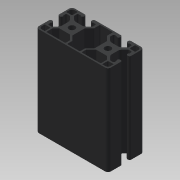
# Autodesk Inventor part: 40-4084-LITE-BLACK-FB
Saved by Autodesk Inventor 2013 (Build 170138000, 138)
## iProperties
Company: 80/20 Inc.
Created: 2014-04-23
Part Number: 40-4084-LITE-BLACK-FB
Material: Generic
Document SubType Name: Modeling
Designer: Ross Bowman
Density: 1 g/cm^3
Engineer: Ross Bowman
Catalog Web Link: 8020.net
Vendor: 80/20 Inc.
Material: 6105-T5 Aluminum
Author: Ross Bowman
Keywords: 80/20 , 8020 , T-Slot , Extrusion
Autodesk Inventor part; units mm, degrees
ref_plane "YZ Plane" through (0, 0, 0) normal (1, 0, 0) x (0, 1, 0)
ref_plane "XZ Plane" through (0, 0, 0) normal (0, 1, 0) x (-1, 0, 0)
ref_plane "XY Plane" through (0, 0, 0) normal (0, 0, 1) x (1, 0, 0)
sketch "Sketch1" plane through (0, 0, 0) normal (0, 0, 1) x (1, 0, 0)
  arc A0 (32.3165, 18.3492) -> (31.9365, 17.9693) centre (32.3165, 17.9693) ccw
  line L0 (35.5555, 18.3492) -> (32.3165, 18.3492)
  arc A1 (38.3495, 15.5552) -> (35.5555, 18.3492) centre (35.5555, 15.5552) ccw
  line L1 (38.3495, 12.3165) -> (38.3495, 15.5552)
  arc A2 (37.9695, 11.9365) -> (38.3495, 12.3165) centre (37.9695, 12.3165) ccw
  line L2 (33.2063, 11.9365) -> (37.9695, 11.9365)
  arc A3 (31.9365, 13.2063) -> (33.2063, 11.9365) centre (33.2063, 13.2063) ccw
  line L3 (31.9365, 17.9693) -> (31.9365, 13.2063)
  arc A4 (35.5555, -18.3492) -> (38.3495, -15.5552) centre (35.5555, -15.5552) ccw
  line L4 (32.3165, -18.3492) -> (35.5555, -18.3492)
  arc A5 (31.9365, -17.9693) -> (32.3165, -18.3492) centre (32.3165, -17.9693) ccw
  line L5 (31.9365, -13.2063) -> (31.9365, -17.9693)
  arc A6 (33.2063, -11.9365) -> (31.9365, -13.2063) centre (33.2063, -13.2063) ccw
  line L6 (37.9695, -11.9365) -> (33.2063, -11.9365)
  arc A7 (38.3495, -12.3165) -> (37.9695, -11.9365) centre (37.9695, -12.3165) ccw
  line L7 (38.3495, -15.5552) -> (38.3495, -12.3165)
  arc A8 (-35.5555, 18.3492) -> (-38.3495, 15.5552) centre (-35.5555, 15.5552) ccw
  line L8 (-32.3165, 18.3492) -> (-35.5555, 18.3492)
  arc A9 (-31.9365, 17.9693) -> (-32.3165, 18.3492) centre (-32.3165, 17.9693) ccw
  line L9 (-31.9365, 13.2063) -> (-31.9365, 17.9693)
  arc A10 (-33.2063, 11.9365) -> (-31.9365, 13.2063) centre (-33.2063, 13.2063) ccw
  line L10 (-37.9695, 11.9365) -> (-33.2063, 11.9365)
  arc A11 (-38.3495, 12.3165) -> (-37.9695, 11.9365) centre (-37.9695, 12.3165) ccw
  line L11 (-38.3495, 15.5552) -> (-38.3495, 12.3165)
  circle A12 centre (-20, 0) radius 3.3778
  circle A13 centre (20, 0) radius 3.3778
  arc A14 (-32.3165, -18.3492) -> (-31.9365, -17.9693) centre (-32.3165, -17.9693) ccw
  line L12 (-35.5555, -18.3492) -> (-32.3165, -18.3492)
  arc A15 (-38.3495, -15.5552) -> (-35.5555, -18.3492) centre (-35.5555, -15.5552) ccw
  line L13 (-38.3495, -12.3165) -> (-38.3495, -15.5552)
  arc A16 (-37.9695, -11.9365) -> (-38.3495, -12.3165) centre (-37.9695, -12.3165) ccw
  line L14 (-33.2063, -11.9365) -> (-37.9695, -11.9365)
  arc A17 (-31.9365, -13.2063) -> (-33.2063, -11.9365) centre (-33.2063, -13.2063) ccw
  line L15 (-31.9365, -17.9693) -> (-31.9365, -13.2063)
  arc A18 (6.3492, -18.3492) -> (7.1111, -17.5873) centre (6.3492, -17.5873) ccw
  line L16 (-6.3492, -18.3492) -> (6.3492, -18.3492)
  arc A19 (-7.1111, -17.5873) -> (-6.3492, -18.3492) centre (-6.3492, -17.5873) ccw
  line L17 (-7.1111, -12.8453) -> (-7.1111, -17.5873)
  arc A20 (-7.1111, -12.8453) -> (-7.3343, -12.3066) centre (-7.873, -12.8453) ccw
  line L18 (-12.0943, -7.5465) -> (-7.3343, -12.3066)
  arc A21 (-12.3175, -7.0078) -> (-12.0943, -7.5465) centre (-11.5556, -7.0078) ccw
  line L19 (-12.3175, 6.1099) -> (-12.3175, -7.0078)
  arc A22 (-12.0943, 6.6486) -> (-12.3175, 6.1099) centre (-11.5556, 6.1099) ccw
  line L20 (-7.3978, 11.3452) -> (-12.0943, 6.6486)
  arc A23 (-7.3978, 11.3452) -> (-7.1746, 11.8839) centre (-7.9365, 11.8839) ccw
  line L21 (-7.1746, 17.5873) -> (-7.1746, 11.8839)
  arc A24 (-6.4127, 18.3492) -> (-7.1746, 17.5873) centre (-6.4127, 17.5873) ccw
  line L22 (6.4127, 18.3492) -> (-6.4127, 18.3492)
  arc A25 (7.1746, 17.5873) -> (6.4127, 18.3492) centre (6.4127, 17.5873) ccw
  line L23 (7.1746, 11.8839) -> (7.1746, 17.5873)
  arc A26 (7.1746, 11.8839) -> (7.3978, 11.3452) centre (7.9365, 11.8839) ccw
  line L24 (12.0943, 6.6486) -> (7.3978, 11.3452)
  arc A27 (12.3175, 6.1099) -> (12.0943, 6.6486) centre (11.5556, 6.1099) ccw
  line L25 (12.3175, -7.0078) -> (12.3175, 6.1099)
  arc A28 (12.0943, -7.5465) -> (12.3175, -7.0078) centre (11.5556, -7.0078) ccw
  line L26 (7.3343, -12.3066) -> (12.0943, -7.5465)
  arc A29 (7.3343, -12.3066) -> (7.1111, -12.8453) centre (7.873, -12.8453) ccw
  line L27 (7.1111, -17.5873) -> (7.1111, -12.8453)
  arc A30 (-26.1099, -7.6825) -> (-26.6486, -7.9057) centre (-26.1099, -8.4444) ccw
  line L28 (-14.9676, -7.6825) -> (-26.1099, -7.6825)
  arc A31 (-14.4289, -7.9057) -> (-14.9676, -7.6825) centre (-14.9676, -8.4444) ccw
  line L29 (-9.239, -13.0955) -> (-14.4289, -7.9057)
  arc A32 (-9.0159, -13.6343) -> (-9.239, -13.0955) centre (-9.7778, -13.6343) ccw
  line L30 (-9.0159, -17.5873) -> (-9.0159, -13.6343)
  arc A33 (-9.7778, -18.3492) -> (-9.0159, -17.5873) centre (-9.7778, -17.5873) ccw
  line L31 (-29.5238, -18.3492) -> (-9.7778, -18.3492)
  arc A34 (-30.2857, -17.5873) -> (-29.5238, -18.3492) centre (-29.5238, -17.5873) ccw
  line L32 (-30.2857, -11.8584) -> (-30.2857, -17.5873)
  arc A35 (-30.0626, -11.3196) -> (-30.2857, -11.8584) centre (-29.5238, -11.8584) ccw
  line L33 (-26.6486, -7.9057) -> (-30.0626, -11.3196)
  arc A36 (9.0159, -17.5873) -> (9.7778, -18.3492) centre (9.7778, -17.5873) ccw
  line L34 (9.0159, -13.6343) -> (9.0159, -17.5873)
  arc A37 (9.239, -13.0955) -> (9.0159, -13.6343) centre (9.7778, -13.6343) ccw
  line L35 (14.4289, -7.9057) -> (9.239, -13.0955)
  arc A38 (14.9676, -7.6825) -> (14.4289, -7.9057) centre (14.9676, -8.4444) ccw
  line L36 (26.1099, -7.6825) -> (14.9676, -7.6825)
  arc A39 (26.6486, -7.9057) -> (26.1099, -7.6825) centre (26.1099, -8.4444) ccw
  line L37 (30.0626, -11.3196) -> (26.6486, -7.9057)
  arc A40 (30.2857, -11.8584) -> (30.0626, -11.3196) centre (29.5238, -11.8584) ccw
  line L38 (30.2857, -17.5873) -> (30.2857, -11.8584)
  arc A41 (29.5238, -18.3492) -> (30.2857, -17.5873) centre (29.5238, -17.5873) ccw
  line L39 (9.7778, -18.3492) -> (29.5238, -18.3492)
  arc A42 (15.9365, 18.4254) -> (14.3619, 20) centre (14.3619, 18.4254) ccw
  line L40 (14.3619, 20) -> (-14.3619, 20)
  arc A43 (-14.3619, 20) -> (-15.9365, 18.4254) centre (-14.3619, 18.4254) ccw
  line L41 (-15.9365, 18.4254) -> (-15.9365, 17.5111)
  arc A44 (-15.9365, 17.5111) -> (-14.3619, 15.9365) centre (-14.3619, 17.5111) ccw
  line L42 (-14.3619, 15.9365) -> (-13.6554, 15.9365)
  arc A45 (-13.6554, 15.9365) -> (-13.2757, 16.3032) centre (-13.6554, 16.3165) ccw
  line L43 (-13.2757, 16.3032) -> (-13.2747, 16.3317)
  arc A46 (-12.895, 16.6984) -> (-13.2747, 16.3317) centre (-12.895, 16.3185) ccw
  line L44 (-12.895, 16.6984) -> (-10.9841, 16.6984)
  arc A47 (-9.7143, 15.4286) -> (-10.9841, 16.6984) centre (-10.9841, 15.4286) ccw
  line L45 (-9.7143, 15.4286) -> (-9.7143, 12.9885)
  arc A48 (-9.9746, 12.3599) -> (-9.7143, 12.9885) centre (-10.6032, 12.9885) ccw
  line L46 (-9.9746, 12.3599) -> (-13.261, 9.0736)
  arc A49 (-16.6192, 7.6825) -> (-13.261, 9.0736) centre (-16.6192, 12.4317) ccw
  line L47 (-16.6192, 7.6825) -> (-23.3808, 7.6825)
  arc A50 (-26.739, 9.0736) -> (-23.3808, 7.6825) centre (-23.3808, 12.4317) ccw
  line L48 (-26.739, 9.0736) -> (-30.0254, 12.3599)
  arc A51 (-30.2857, 12.9885) -> (-30.0254, 12.3599) centre (-29.3968, 12.9885) ccw
  line L49 (-30.2857, 12.9885) -> (-30.2857, 15.4286)
  arc A52 (-29.0159, 16.6984) -> (-30.2857, 15.4286) centre (-29.0159, 15.4286) ccw
  line L50 (-29.0159, 16.6984) -> (-26.7381, 16.6984)
  line L51 (-26.7381, 16.6984) -> (-26.7115, 15.9365)
  line L52 (-26.7115, 15.9365) -> (-25.6381, 15.9365)
  arc A53 (-25.6381, 15.9365) -> (-24.0635, 17.5111) centre (-25.6381, 17.5111) ccw
  line L53 (-24.0635, 17.5111) -> (-24.0635, 18.4254)
  arc A54 (-24.0635, 18.4254) -> (-25.6381, 20) centre (-25.6381, 18.4254) ccw
  line L54 (-25.6381, 20) -> (-36.8254, 20)
  arc A55 (-36.8254, 20) -> (-40, 16.8252) centre (-36.8254, 16.8254) ccw
  line L55 (-40, 16.8252) -> (-39.9994, 5.6381)
  arc A56 (-39.9994, 5.6381) -> (-38.4248, 4.0635) centre (-38.4248, 5.6381) ccw
  line L56 (-38.4248, 4.0635) -> (-37.5105, 4.0635)
  arc A57 (-37.5105, 4.0635) -> (-35.9359, 5.6381) centre (-37.5105, 5.6381) ccw
  line L57 (-35.9359, 5.6381) -> (-35.9359, 6.3092)
  arc A58 (-35.9359, 6.3092) -> (-36.3026, 6.689) centre (-36.3158, 6.3092) ccw
  line L58 (-36.3026, 6.689) -> (-36.3311, 6.69)
  arc A59 (-36.6978, 7.0697) -> (-36.3311, 6.69) centre (-36.3178, 7.0697) ccw
  line L59 (-36.6978, 7.0697) -> (-36.6978, 9.0159)
  arc A60 (-35.428, 10.2857) -> (-36.6978, 9.0159) centre (-35.428, 9.0159) ccw
  line L60 (-35.428, 10.2857) -> (-32.9885, 10.2857)
  arc A61 (-32.3599, 10.0254) -> (-32.9885, 10.2857) centre (-32.9885, 9.3968) ccw
  line L61 (-32.3599, 10.0254) -> (-29.0736, 6.739)
  arc A62 (-27.6825, 3.3808) -> (-29.0736, 6.739) centre (-32.4317, 3.3808) ccw
  line L62 (-27.6825, 3.3808) -> (-27.6825, -3.3808)
  arc A63 (-29.0736, -6.739) -> (-27.6825, -3.3808) centre (-32.4317, -3.3808) ccw
  line L63 (-29.0736, -6.739) -> (-32.3599, -10.0254)
  arc A64 (-32.9885, -10.2857) -> (-32.3599, -10.0254) centre (-32.9885, -9.3968) ccw
  line L64 (-32.9885, -10.2857) -> (-35.4286, -10.2857)
  arc A65 (-36.6984, -9.0159) -> (-35.4286, -10.2857) centre (-35.4286, -9.0159) ccw
  line L65 (-36.6984, -9.0159) -> (-36.6984, -7.105)
  arc A66 (-36.3175, -6.7251) -> (-36.6984, -7.105) centre (-36.3185, -7.105) ccw
  arc A67 (-36.3175, -6.7251) -> (-35.9365, -6.3451) centre (-36.3165, -6.3451) ccw
  line L66 (-35.9365, -6.3451) -> (-35.9365, -5.6381)
  arc A68 (-35.9365, -5.6381) -> (-37.5111, -4.0635) centre (-37.5111, -5.6381) ccw
  line L67 (-37.5111, -4.0635) -> (-38.4254, -4.0635)
  arc A69 (-38.4254, -4.0635) -> (-40, -5.6381) centre (-38.4254, -5.6381) ccw
  line L68 (-40, -5.6381) -> (-40, -16.8254)
  arc A70 (-40, -16.8254) -> (-36.8254, -20) centre (-36.8254, -16.8254) ccw
  line L69 (-36.8254, -20) -> (36.8254, -20)
  arc A71 (36.8254, -20) -> (40, -16.8254) centre (36.8254, -16.8254) ccw
  line L70 (40, -16.8254) -> (40, -5.6381)
  arc A72 (40, -5.6381) -> (38.4254, -4.0635) centre (38.4254, -5.6381) ccw
  line L71 (38.4254, -4.0635) -> (37.5111, -4.0635)
  arc A73 (37.5111, -4.0635) -> (35.9365, -5.6381) centre (37.5111, -5.6381) ccw
  line L72 (35.9365, -5.6381) -> (35.9365, -6.3446)
  arc A74 (35.9365, -6.3446) -> (36.3032, -6.7243) centre (36.3165, -6.3446) ccw
  line L73 (36.3032, -6.7243) -> (36.3317, -6.7253)
  arc A75 (36.6984, -7.105) -> (36.3317, -6.7253) centre (36.3185, -7.105) ccw
  line L74 (36.6984, -7.105) -> (36.6984, -9.0159)
  arc A76 (35.4286, -10.2857) -> (36.6984, -9.0159) centre (35.4286, -9.0159) ccw
  line L75 (35.4286, -10.2857) -> (32.9885, -10.2857)
  arc A77 (32.3599, -10.0254) -> (32.9885, -10.2857) centre (32.9885, -9.3968) ccw
  line L76 (32.3599, -10.0254) -> (29.0736, -6.739)
  arc A78 (27.6825, -3.3808) -> (29.0736, -6.739) centre (32.4317, -3.3808) ccw
  line L77 (27.6825, -3.3808) -> (27.6825, 3.3808)
  arc A79 (29.0736, 6.739) -> (27.6825, 3.3808) centre (32.4317, 3.3808) ccw
  line L78 (29.0736, 6.739) -> (32.3599, 10.0254)
  arc A80 (32.9885, 10.2857) -> (32.3599, 10.0254) centre (32.9885, 9.3968) ccw
  line L79 (32.9885, 10.2857) -> (35.4286, 10.2857)
  arc A81 (36.6984, 9.0159) -> (35.4286, 10.2857) centre (35.4286, 9.0159) ccw
  line L80 (36.6984, 9.0159) -> (36.6984, 7.105)
  arc A82 (36.3317, 6.7253) -> (36.6984, 7.105) centre (36.3185, 7.105) ccw
  line L81 (36.3317, 6.7253) -> (36.3032, 6.7243)
  arc A83 (36.3032, 6.7243) -> (35.9365, 6.3446) centre (36.3165, 6.3446) ccw
  line L82 (35.9365, 6.3446) -> (35.9365, 5.5746)
  arc A84 (35.9365, 5.5746) -> (37.5022, 4.0635) centre (37.4965, 5.6242) ccw
  line L83 (37.5022, 4.0635) -> (38.4165, 4.0635)
  arc A85 (38.4165, 4.0635) -> (40, 5.5746) centre (38.4087, 5.6569) ccw
  line L84 (40, 5.5746) -> (40, 16.8254)
  arc A86 (40, 16.8254) -> (36.8254, 20) centre (36.8254, 16.8254) ccw
  line L85 (36.8254, 20) -> (25.6381, 20)
  arc A87 (25.6381, 20) -> (24.0635, 18.4254) centre (25.6381, 18.4254) ccw
  line L86 (24.0635, 18.4254) -> (24.0635, 17.5111)
  arc A88 (24.0635, 17.5111) -> (25.6381, 15.9365) centre (25.6381, 17.5111) ccw
  line L87 (25.6381, 15.9365) -> (26.3446, 15.9365)
  arc A89 (26.3446, 15.9365) -> (26.7243, 16.3032) centre (26.3446, 16.3165) ccw
  line L88 (26.7243, 16.3032) -> (26.7253, 16.3317)
  arc A90 (27.105, 16.6984) -> (26.7253, 16.3317) centre (27.105, 16.3185) ccw
  line L89 (27.105, 16.6984) -> (29.0159, 16.6984)
  arc A91 (30.2857, 15.4286) -> (29.0159, 16.6984) centre (29.0159, 15.4286) ccw
  line L90 (30.2857, 15.4286) -> (30.2857, 12.9885)
  arc A92 (30.0254, 12.3599) -> (30.2857, 12.9885) centre (29.3968, 12.9885) ccw
  line L91 (30.0254, 12.3599) -> (26.739, 9.0736)
  arc A93 (23.3808, 7.6825) -> (26.739, 9.0736) centre (23.3808, 12.4317) ccw
  line L92 (23.3808, 7.6825) -> (16.6192, 7.6825)
  arc A94 (13.261, 9.0736) -> (16.6192, 7.6825) centre (16.6192, 12.4317) ccw
  line L93 (13.261, 9.0736) -> (9.9746, 12.3599)
  arc A95 (9.7143, 12.9885) -> (9.9746, 12.3599) centre (10.6032, 12.9885) ccw
  line L94 (9.7143, 12.9885) -> (9.7143, 15.4346)
  arc A96 (10.9875, 16.7044) -> (9.7143, 15.4346) centre (10.9841, 15.4346) ccw
  line L95 (10.9875, 16.7044) -> (12.896, 16.6994)
  arc A97 (13.2747, 16.3327) -> (12.896, 16.6994) centre (12.895, 16.3194) ccw
  line L96 (13.2747, 16.3327) -> (13.2757, 16.3032)
  arc A98 (13.2757, 16.3032) -> (13.6554, 15.9365) centre (13.6554, 16.3165) ccw
  line L97 (13.6554, 15.9365) -> (14.3619, 15.9365)
  arc A99 (14.3619, 15.9365) -> (15.9365, 17.5111) centre (14.3619, 17.5111) ccw
  line L98 (15.9365, 17.5111) -> (15.9365, 18.4254)
  point P0 (0, 0)
  constraints: 198 end point, 196 point on circle, 100 centre point
extrude "Extrusion1" add sketch "Sketch1" against normal blind 100
body "Solid1"
